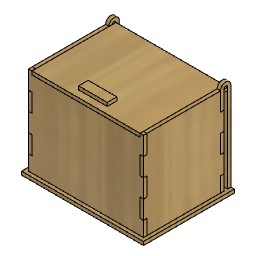
MyBox (Autodesk Fusion 360 design; units mm, degrees)
Autodesk Fusion 360 part; units mm, degrees
note: some values were not read from the file. Set by a fixed rule: which sketch regions a step uses.
sketch "Sketch1" plane through (0, 0, 0) normal (0, 1, 0) x (1, 0, 0) in component "front"
  line L0 (0, 0) -> (100, 0)
  line L1 (100, 0) -> (100, -80)
  line L2 (100, -80) -> (0, -80)
  line L3 (0, -80) -> (0, 0)
  line L4 (0, -3) -> (100, -3) construction
  line L5 (3, 0) -> (3, -80) construction
  line L6 (0, -64) -> (3, -64)
  line L7 (3, -64) -> (3, -48)
  line L8 (3, -48) -> (0, -48)
  line L9 (0, -48) -> (0, -64)
  line L10 (0, -32) -> (3, -32)
  line L11 (3, -32) -> (3, -16)
  line L12 (3, -16) -> (0, -16)
  line L13 (0, -16) -> (0, -32)
  line L14 (20, 0) -> (40, 0)
  line L15 (40, 0) -> (40, -3)
  line L16 (40, -3) -> (20, -3)
  line L17 (20, -3) -> (20, 0)
  line L18 (60, 0) -> (80, 0)
  line L19 (80, 0) -> (80, -3)
  line L20 (80, -3) -> (60, -3)
  line L21 (60, -3) -> (60, 0)
  line L22 (50, -80) -> (50, 0) construction
  line L23 (100, -48) -> (100, -64)
  line L24 (97, -16) -> (100, -16)
  line L25 (100, -64) -> (97, -64)
  line L26 (100, -32) -> (97, -32)
  line L27 (100, -16) -> (100, -32)
  line L28 (97, -64) -> (97, -48)
  line L29 (97, -32) -> (97, -16)
  line L30 (97, -48) -> (100, -48)
  line L31 (97, 0) -> (97, -80) construction
  line L32 (3, -80) -> (97, -80)
  line L33 (97, -80) -> (97, -77)
  line L34 (97, -77) -> (3, -77)
  line L35 (3, -77) -> (3, -80)
  point P0 (100, -80)
  dimension "d7" = 80
  dimension "d8" = 100
  dimension "d10" = 3
  dimension "d11" = 3
  dimension "d12" = 16
  dimension "d13" = 16
  dimension "d14" = 16
  dimension "d15" = 16
  dimension "d16" = 20
  dimension "d17" = 20
  dimension "d18" = 20
  dimension "d19" = 20
  dimension "d41" = 3
  constraint horizontal L0
  constraint vertical L1
  constraint horizontal L2
  constraint vertical L3
  constraint coincident L0.start L3.end
  constraint coincident L3 L4.start
  constraint coincident L1 L4.end
  constraint coincident L0 L5.start
  constraint coincident L2 L5.end
  constraint vertical L5
  constraint horizontal L4
  constraint horizontal L6
  constraint vertical L7
  constraint horizontal L8
  constraint vertical L9
  constraint coincident L5 L7.end
  constraint coincident L3 L6.start
  constraint horizontal L10
  constraint vertical L11
  constraint horizontal L12
  constraint vertical L13
  constraint coincident L5 L11.end
  constraint coincident L3 L10.start
  constraint horizontal L14
  constraint vertical L15
  constraint horizontal L16
  constraint vertical L17
  constraint coincident L4 L15.end
  constraint coincident L0 L14.start
  constraint horizontal L18
  constraint vertical L19
  constraint horizontal L20
  constraint vertical L21
  constraint coincident L4 L19.end
  constraint coincident L0 L18.start
  constraint midpoint L2 L22.start
  constraint midpoint L0 L22.end
  constraint symmetric L2.end L22 P0
  constraint symmetric L5.start L22 L31.start
  constraint symmetric L5.end L22 L31.end
  constraint symmetric L6.start L22 L23.end
  constraint symmetric L6.end L22 L25.end
  constraint symmetric L7.end L22 L28.end
  constraint symmetric L8.end L22 L23.start
  constraint symmetric L10.start L22 L26.start
  constraint symmetric L10.end L22 L26.end
  constraint symmetric L11.end L22 L24.start
  constraint symmetric L12.end L22 L24.end
  constraint horizontal L32
  constraint vertical L33
  constraint horizontal L34
  constraint vertical L35
  constraint coincident L31 L33.end
  measures "d7" distance of L0.start L2.end
  measures "d8" distance of L0.start L0.end
  measures "d10" distance of L0 L4
  measures "d11" distance of L3 L5
  measures "d12" distance of L2 L6
  measures "d13" distance of L6 L8
  measures "d14" distance of L8 L10
  measures "d15" distance of L10 L12
  measures "d16" distance of L3 L17
  measures "d17" distance of L15 L17
  measures "d18" distance of L15 L21
  measures "d19" distance of L19 L21
  measures "d41" distance of L32 L34
extrude "Extrude1" add sketch "Sketch1" along normal blind 3 contours L0 L1 L2 L3 L6 L7 L8 L10 L11 L12 L15 L16 L17 L19 L20 L21 L24 L25 L26 L28 L29 L30 L33 L34 L35 makes body 1 in component "front"
sketch "Sketch1 (2)" plane through (0, 0, 0) normal (-1, 0, 0) x (0, -1, 0) in component "left"
  line L0 (0, 0) -> (0, 16)
  line L1 (0, 16) -> (-3, 16)
  line L2 (-3, 16) -> (-3, 0)
  line L3 (-3, 0) -> (0, 0)
  line L4 (0, 0) -> (-70, 0)
  line L5 (-70, 0) -> (-70, 80)
  line L6 (-70, 80) -> (0, 80)
  line L7 (0, 80) -> (0, 0)
  line L8 (0, 80) -> (-3, 80)
  line L9 (0, 3) -> (-70, 3) construction
  line L10 (-67, 80) -> (-67, 0) construction
  line L11 (-70, 64) -> (-67, 64)
  line L12 (-67, 64) -> (-67, 48)
  line L13 (-67, 48) -> (-70, 48)
  line L14 (-70, 48) -> (-70, 64)
  line L15 (-70, 32) -> (-67, 32)
  line L16 (-67, 32) -> (-67, 16)
  line L17 (-67, 16) -> (-70, 16)
  line L18 (-70, 16) -> (-70, 32)
  line L19 (-56, 3) -> (-42, 3)
  line L20 (-42, 3) -> (-42, 0)
  line L21 (-42, 0) -> (-56, 0)
  line L22 (-56, 0) -> (-56, 3)
  line L23 (-28, 3) -> (-14, 3)
  line L24 (-14, 3) -> (-14, 0)
  line L25 (-14, 0) -> (-28, 0)
  line L26 (-28, 0) -> (-28, 3)
  line L27 (-35, 80) -> (-35, 0) construction
  line L28 (-3, 48) -> (0, 48)
  line L29 (0, 64) -> (-3, 64)
  line L30 (0, 48) -> (0, 64)
  line L31 (-3, 64) -> (-3, 48)
  line L32 (-3, 32) -> (-3, 16)
  line L33 (-3, 16) -> (0, 16)
  line L34 (0, 16) -> (0, 32)
  line L35 (0, 32) -> (-3, 32)
  line L36 (-3, 80) -> (-3, 0) construction
  dimension "d22" = 70
  dimension "d23" = 3
  dimension "d24" = 3
  dimension "d25" = 16
  dimension "d26" = 16
  dimension "d27" = 16
  dimension "d28" = 16
  dimension "d29" = 14
  dimension "d30" = 14
  dimension "d31" = 14
  dimension "d32" = 14
  constraint horizontal L4
  constraint vertical L5
  constraint horizontal L6
  constraint vertical L7
  constraint collinear L0 L7
  constraint collinear L3 L4
  constraint collinear L6 L8
  constraint coincident L7 L9.start
  constraint coincident L5 L9.end
  constraint perpendicular L5 L9
  constraint coincident L6 L10.start
  constraint coincident L4 L10.end
  constraint perpendicular L4 L10
  constraint horizontal L11
  constraint vertical L12
  constraint horizontal L13
  constraint vertical L14
  constraint coincident L10 L12.end
  constraint coincident L5 L11.start
  constraint horizontal L15
  constraint vertical L16
  constraint horizontal L17
  constraint vertical L18
  constraint coincident L10 L16.end
  constraint coincident L5 L15.start
  constraint horizontal L19
  constraint vertical L20
  constraint horizontal L21
  constraint vertical L22
  constraint coincident L4 L20.end
  constraint coincident L9 L19.start
  constraint horizontal L23
  constraint vertical L24
  constraint horizontal L25
  constraint vertical L26
  constraint coincident L4 L24.end
  constraint coincident L9 L23.start
  constraint midpoint L6 L27.start
  constraint midpoint L4 L27.end
  constraint symmetric L10.start L27 L8.end
  constraint symmetric L10.end L27 L2.end
  constraint symmetric L11.start L27 L29.start
  constraint symmetric L11.end L27 L29.end
  constraint symmetric L12.end L27 L28.start
  constraint symmetric L13.end L27 L28.end
  constraint symmetric L15.start L27 L34.end
  constraint symmetric L15.end L27 L32.start
  constraint symmetric L16.end L27 L1.end
  constraint symmetric L17.end L27 L0.end
  measures "d22" distance of L0.start L4.end
  measures "d23" distance of L4 L9
  measures "d24" distance of L5 L10
  measures "d25" distance of L6 L11
  measures "d26" distance of L11 L13
  measures "d27" distance of L13 L15
  measures "d28" distance of L15 L17
  measures "d29" distance of L5 L22
  measures "d30" distance of L20 L22
  measures "d31" distance of L20 L26
  measures "d32" distance of L24 L26
extrude "Extrude1'" add sketch "Sketch1 (2)" against normal blind 3 separate body contours L0 L1 L2 L3 L4 L7 L33 | L1 L7 L32 L33 L34 L35 | L2 L4 L5 L6 L7 L8 L11 L12 L13 L15 L16 L17 L19 L20 L22 L23 L24 L26 L28 L29 L31 L32 L35 | L7 L28 L29 L30 L31 | L5 L15 L16 L17 L18 | L5 L11 L12 L13 L14 makes body 2 in component "left"
ref_plane "WorkPlane1" through (50, 35, 40) normal (0, -1, 0) x (-1, 0, 0)
ref_plane "WorkPlane2" through (50, 35, 40) normal (-1, 0, 0) x (0, -1, 0)
mirror "MirrorComponent1" about plane through (0, 0, 0) normal (0, 0, 1) of bodies 1 makes body 3 in component "back"
mirror "MirrorComponent2" about plane through (0, 0, 0) normal (0, 0, 1) of bodies 2 makes body 4 in component "right"
combine "Combine1" operation cut target body 2 tool bodies 3 1 body 3 seen with x (1, 0, 0) y (0, -1, 0) z (0, 0, -1) at (0, 70, 0) keep tools in component "left"
combine "Combine1'" operation cut target body 4 tool bodies 3 1 body 3 seen with x (-1, 0, 0) y (0, -1, 0) z (0, 0, 1) at (100, 70, 0) body 1 seen with x (-1, 0, 0) y (0, 1, 0) z (0, 0, -1) at (100, 0, 0) keep tools in component "right"
sketch "Sketch1 (3)" plane through (0, 0, 3) normal (0, 0, -1) x (1, 0, 0) in component "bottom"
  line L0 (40, 0) -> (20, 0)
  line L1 (20, 0) -> (20, -3)
  line L2 (20, -3) -> (40, -3)
  line L3 (40, -3) -> (40, 0)
  line L4 (-3, 3) -> (103, 3)
  line L5 (103, 3) -> (103, -76)
  line L6 (103, -76) -> (-3, -76)
  line L7 (-3, -76) -> (-3, 3)
  line L8 (100, 0) -> (100, -3)
  line L9 (100, 0) -> (97, 0)
  line L10 (97, -3) -> (100, -3)
  line L11 (0, 0) -> (0, -3)
  line L12 (3, 0) -> (0, 0)
  line L13 (3, -3) -> (3, 0)
  line L14 (0, 0) -> (0, -3)
  line L15 (3, -67) -> (3, -3)
  line L16 (0, -3) -> (0, -67)
  line L17 (3, -70) -> (3, -67)
  line L18 (0, -70) -> (3, -70)
  line L19 (0, -67) -> (0, -70)
  line L20 (100, -70) -> (100, -67)
  line L21 (100, -70) -> (97, -70)
  line L22 (0, -70) -> (0, -67)
  line L23 (97, -67) -> (100, -67)
  line L24 (100, 0) -> (97, 0)
  line L25 (100, -3) -> (100, 0)
  line L26 (97, 0) -> (97, -3)
  line L27 (97, -67) -> (97, -3)
  line L28 (97, -67) -> (97, -70)
  line L29 (97, -70) -> (100, -70)
  line L30 (100, -70) -> (100, -67)
  line L31 (100, -3) -> (100, -67)
  line L32 (97, 0) -> (3, 0)
  line L33 (3, -3) -> (97, -3)
  line L34 (3, 0) -> (0, 0)
  line L35 (0, -3) -> (3, -3)
  line L36 (97, -70) -> (3, -70)
  line L37 (3, -67) -> (97, -67)
  line L38 (3, -70) -> (0, -70)
  line L39 (0, -67) -> (3, -67)
  dimension "d35" = 3
  dimension "d36" = 3
  dimension "d37" = 3
  dimension "d38" = 6
  constraint horizontal L4
  constraint vertical L5
  constraint horizontal L6
  constraint vertical L7
  measures "d35" distance of L4 L9
  measures "d36" distance of L7 L16
  measures "d37" distance of L5 L31
  measures "d38" distance of L6 L21
extrude "Extrude1''" add sketch "Sketch1 (3)" along normal blind 3 separate body contours L0 L1 L2 L3 L32 L33 | L3 L26 L32 L33 | L1 L13 L32 L33 | L2 L15 L27 L33 L37 | L8 L9 L10 L24 L25 L26 | L11 L12 L13 L14 L34 L35 | L10 L23 L27 L31 | L15 L16 L35 L39 | L20 L21 L23 L28 L29 L30 | L17 L28 L36 L37 | L17 L18 L19 L22 L38 L39 | L4 L5 L6 L7 makes body 5 in component "bottom"
combine "Combine1''" operation cut target body 5 tool bodies 3 4 1 2 body 3 seen with x (1, 0, 0) y (0, -1, 0) z (0, 0, -1) at (0, 70, 0) body 4 seen with x (-1, 0, 0) y (0, 1, 0) z (0, 0, -1) at (100, 0, 0) keep tools in component "bottom"
sketch "Sketch1 (4)" plane through (0, 0, 77) normal (0, 0, 1) x (-1, 0, 0) in component "top"
  line L0 (-97, -70) -> (-3, -70)
  line L1 (-3, -70) -> (-3, -67)
  line L2 (-3, -67) -> (-97, -67)
  line L3 (-97, -67) -> (-97, -70)
  line L4 (-3, -73) -> (-97, -73)
  line L5 (-97, -73) -> (-97, 0)
  line L6 (-97, 0) -> (-3, 0)
  line L7 (-3, 0) -> (-3, -73)
  line L8 (-3, -67) -> (-3, -3)
  line L9 (-97, -67) -> (-97, -3)
  line L10 (-97, 0) -> (-3, 0)
  dimension "d42" = 3
  constraint horizontal L4
  constraint vertical L5
  constraint horizontal L6
  constraint vertical L7
  constraint collinear L7 L8
  constraint collinear L5 L9
  constraint collinear L6 L10
  measures "d42" distance of L0 L4
extrude "Extrude1'''" add sketch "Sketch1 (4)" along normal blind 3 separate body makes body 6 in component "top"
sketch "Sketch1 (5)" plane through (100, 0, 0) normal (1, 0, 0) x (0, 1, 0) in component "back"
  line L0 (0, -64) -> (0, -80)
  line L1 (0, -80) -> (3, -80)
  line L2 (3, -80) -> (3, -64)
  line L3 (3, -64) -> (0, -64)
  line L4 (-6, -80) -> (-3, -80)
  line L5 (-3, -80) -> (-3, -3)
  line L6 (-3, -3) -> (-6, -3)
  line L7 (-6, -3) -> (-6, -80)
  line L8 (-3, -77) -> (-3, -80)
  line L9 (70, -77) -> (70, -80)
  line L10 (70, -77) -> (-3, -77)
  line L11 (-3, -80) -> (70, -80)
  line L12 (73, -3) -> (-6, -3)
  line L13 (0, 0) -> (0, -16)
  circle A0 centre (-1.5, -80) radius 1.5
  line L14 (0, -80) -> (3, -80)
  line L15 (0, -80) -> (0, -64)
  line L16 (3, -64) -> (3, -80)
  line L17 (0, -64) -> (0, -48)
  line L18 (3, -48) -> (3, -64)
  line L19 (0, -48) -> (0, -32)
  line L20 (3, -32) -> (3, -48)
  line L21 (0, -32) -> (0, -16)
  line L22 (3, -16) -> (3, -32)
  line L23 (0, -16) -> (0, 0)
  line L24 (0, 0) -> (3, 0)
  line L25 (3, 0) -> (3, -16)
  circle A1 centre (-1.5, -80) radius 4.5
  dimension "d45" = 3
  dimension "d50" = 3
  constraint horizontal L4
  constraint vertical L5
  constraint horizontal L6
  constraint vertical L7
  constraint collinear L4 L11
  constraint collinear L6 L12
  constraint coincident L4.end A0
  constraint tangent L5 A0
  constraint coincident L0.end A0
  constraint coincident L4.start A1
  constraint tangent L7 A1
  constraint coincident L1.end A1
  measures "d45" distance of L5 L7
  measures "d50" distance of L0 L5
extrude "Extrude1''''" add sketch "Sketch1 (5)" against normal blind 3 contours L5 L6 L7 L12 A1 | L4 L5 L8 A1 | L1 L4 L11 A0 L14 A1 bodies 3 in component "back"
mirror "Mirror1" about plane through (50, 35, -40) normal (-1, 0, 0) of "Extrude1''''" in component "back"
sketch "Sketch2" plane through (3, 0, 0) normal (1, 0, 0) x (0, 1, 0) in component "back"
  line L0 (0, -77) -> (0, -80)
  arc A0 (-3, -80) -> (0, -80) centre (-1.5, -80) ccw
  line L1 (-3, -80) -> (-3, -3)
  line L2 (-3, -3) -> (-6, -3)
  line L3 (-6, -3) -> (-6, -80)
  arc A1 (-6, -80) -> (3, -80) centre (-1.5, -80) ccw
  line L4 (3, -80) -> (3, -77)
  line L5 (3, -77) -> (0, -77)
  line L6 (-3, -64) -> (-6, -64)
  line L7 (-6, -64) -> (-6, -48)
  line L8 (-6, -48) -> (-3, -48)
  line L9 (-3, -48) -> (-3, -64)
  line L10 (-3, -32) -> (-6, -32)
  line L11 (-6, -32) -> (-6, -16)
  line L12 (-6, -16) -> (-3, -16)
  line L13 (-3, -16) -> (-3, -32)
  line L14 (-6, -80) -> (-3, -80)
  dimension "d51" = 16
  dimension "d52" = 16
  dimension "d53" = 16
  dimension "d54" = 16
  constraint horizontal L6
  constraint vertical L7
  constraint horizontal L8
  constraint vertical L9
  constraint coincident L3 L7.end
  constraint coincident L1 L6.start
  constraint horizontal L10
  constraint vertical L11
  constraint horizontal L12
  constraint vertical L13
  constraint coincident L3 L11.end
  constraint coincident L1 L10.start
  measures "d51" distance of L6 L14
  measures "d52" distance of L6 L8
  measures "d53" distance of L8 L10
  measures "d54" distance of L10 L12
extrude "Extrude2" add sketch "Sketch2" along normal up to near side of body 3 contours L1 L3 L6 L7 L8 L9 | L1 L3 L10 L11 L12 L13 bodies 3 in component "back"
sketch "Sketch2 (2)" plane through (3, 0, 0) normal (-1, 0, 0) x (0, -1, 0) in component "top"
  line L0 (-73, 77) -> (0, 77)
  line L1 (0, 77) -> (0, 80)
  line L2 (0, 80) -> (-73, 80)
  line L3 (-73, 80) -> (-73, 77)
  line L4 (-73, 77) -> (-73, 80)
  line L5 (-73, 77) -> (0, 77)
  line L6 (0, 80) -> (-73, 80)
  line L7 (0, 77) -> (0, 80)
  line L8 (-73, 80) -> (-70.0137, 77) construction
  line L9 (-70.0137, 80) -> (-73, 77) construction
  circle A0 centre (-71.5069, 78.5) radius 1.475
  dimension "d57" = 2.95
  constraint coincident L2.end L3.start
  constraint coincident L5 L8.end
  constraint coincident L6 L9.start
  constraint coincident L0.start L3.end
  constraint midpoint L9 A0.centre
  measures "d57" diameter of A0
extrude "Extrude2'" add sketch "Sketch2 (2)" along normal blind 3 contours A0 bodies 6 in component "top"
mirror "Mirror1'" about plane through (50, 35, 40) normal (-1, 0, 0) of "Extrude2'" in component "top"
sketch "Sketch3" plane through (0, 0, 80) normal (0, 0, 1) x (-1, 0, 0) in component "top"
  line L0 (-3, -73) -> (-3, 0)
  line L1 (-3, 0) -> (-97, 0)
  line L2 (-97, 0) -> (-97, -73)
  line L3 (-97, -73) -> (-3, -73)
  line L4 (-50, -73) -> (-50, 0) construction
  line L5 (-37.5, -6) -> (-62.5, -6)
  line L6 (-62.5, -6) -> (-62.5, -14.3333)
  line L7 (-62.5, -14.3333) -> (-37.5, -14.3333)
  line L8 (-37.5, -14.3333) -> (-37.5, -6)
  line L9 (-50, -14.3333) -> (-50, -6) construction
  dimension "d63" = 8.3333
  dimension "d64" = 25
  dimension "d65" = 6
  constraint midpoint L3 L4.start
  constraint midpoint L1 L4.end
  constraint horizontal L5
  constraint vertical L6
  constraint horizontal L7
  constraint vertical L8
  constraint midpoint L7 L9.start
  constraint midpoint L5 L9.end
  constraint collinear L4 L9
  measures "d63" distance of L5.end L6.end
  measures "d64" distance of L6.end L7.end
  measures "d65" distance of L1 L5
extrude "Extrude3" add sketch "Sketch3" along normal blind 3 contours L5 L6 L7 L8 bodies 6 in component "top"
component "front" placed x (1, 0, 0) y (0, 1, 0) z (0, 0, 1) at (0, 0, 0)
component "left" placed x (1, 0, 0) y (0, 1, 0) z (0, 0, 1) at (0, 0, 0)
component "bottom" placed x (1, 0, 0) y (0, 1, 0) z (0, 0, 1) at (0, 0, 0)
component "back" placed x (1, 0, 0) y (0, -1, 0) z (0, 0, -1) at (0, 70, 0)
component "right" placed x (-1, 0, 0) y (0, 1, 0) z (0, 0, -1) at (100, 0, 0)
component "top" placed x (1, 0, 0) y (0, 1, 0) z (0, 0, 1) at (0, 0, 0)
equation "length = 100 mm"
equation "height = 80 mm"
equation "width = 70 mm"
equation "ntabs_h = 5"
equation "ntabs_w = 5"
equation "ntabs_l = 5"
equation "d7 = height"
equation "d8 = length"
equation "thickness = 3 mm"
equation "d10 = thickness"
equation "d11 = thickness"
equation "d12 = height / ntabs_h"
equation "d13 = d12"
equation "d14 = d12"
equation "d15 = d12"
equation "d16 = length / ntabs_l"
equation "d17 = d16"
equation "d18 = d16"
equation "d19 = d16"
equation "d20 = thickness"
equation "d22 = width"
equation "d23 = thickness"
equation "d24 = thickness"
equation "d25 = height / ntabs_h"
equation "d26 = d25"
equation "d27 = d25"
equation "d28 = d25"
equation "d29 = width / ntabs_w"
equation "d30 = d29"
equation "d31 = d29"
equation "d32 = d29"
equation "d33 = -thickness"
equation "d35 = thickness"
equation "d36 = thickness"
equation "d37 = thickness"
equation "d38 = 2 * thickness"
equation "d39 = thickness"
equation "d41 = thickness"
equation "d42 = thickness"
equation "d43 = thickness"
equation "d45 = thickness"
equation "d47 = -thickness"
equation "d50 = thickness"
equation "d51 = height / ntabs_h"
equation "d52 = d51"
equation "d53 = d51"
equation "d54 = d51"
equation "d57 = thickness - 0.05 mm"
equation "d58 = thickness"
equation "handlelen = ( 1 / 4 ) * length"
equation "handleht = ( 1 / 3 ) * handlelen"
equation "d63 = handleht"
equation "d64 = handlelen"
equation "d65 = 2 * thickness"
equation "d66 = thickness"
